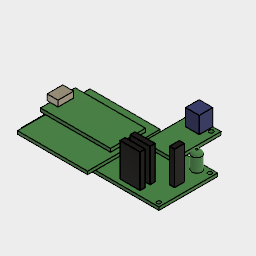
bike_announce_case (Autodesk Fusion 360 archive; units mm, degrees)
design "PCB"
Autodesk Fusion 360 part; units mm, degrees
sketch "Sketch1" plane through (0, 0, 0) normal (0, 0, 1) x (1, 0, 0)
  line L0 (0, 0) -> (70, 0)
  line L1 (70, 0) -> (70, 30)
  line L2 (70, 30) -> (0, 30)
  line L3 (0, 30) -> (0, 0)
  line L4 (0, 15) -> (70, 15) construction
  line L5 (35, 30) -> (35, 0) construction
  circle A0 centre (2, 2) radius 1
  circle A1 centre (2, 28) radius 1
  circle A2 centre (68, 28) radius 1
  circle A3 centre (68, 2) radius 1
  dimension "d1" = 70
  dimension "d2" = 30
  dimension "d22" = 2
  dimension "d23" = 2
  dimension "d24" = 2
  measures "d1" distance of L1.end L2.end
  measures "d2" distance of L0.start L2.end
  measures "d22" diameter of A0
  measures "d23" distance of L0 A0.centre
  measures "d24" distance of L3 A0.centre
extrude "Extrude1" add sketch "Sketch1" along normal blind 1.6 makes body 1
sketch "Sketch5" plane through (0, 0, 1.6) normal (0, 0, 1) x (-1, 0, 0)
  circle A0 centre (-68, -2) radius 1
  circle A1 centre (-2, -2) radius 1
  circle A2 centre (-68, -28) radius 1
  circle A3 centre (-2, -28) radius 1
  line L0 (0, -30) -> (0, 0)
  line L1 (0, 0) -> (-70, 0)
  line L2 (-70, 0) -> (-70, -30)
  line L3 (-70, -30) -> (0, -30)
  line L4 (-47.75, -10.08) -> (-58, -10.08)
  line L5 (-58, -10.08) -> (-58, -7.48)
  line L6 (-58, -7.48) -> (-47.75, -7.48)
  line L7 (-47.75, -7.48) -> (-47.75, -10.08)
  line L8 (-47.75, -5) -> (-58, -5)
  line L9 (-58, -5) -> (-58, -2.4)
  line L10 (-58, -2.4) -> (-47.75, -2.4)
  line L11 (-47.75, -2.4) -> (-47.75, -5)
  line L12 (-58, -3.7) -> (-47.75, -3.7) construction
  line L13 (-47.75, -8.78) -> (-58, -8.78) construction
  line L14 (-62.9, -17.55) -> (-65.5, -17.55)
  line L15 (-65.5, -17.55) -> (-65.5, -12.45)
  line L16 (-65.5, -12.45) -> (-62.9, -12.45)
  line L17 (-62.9, -12.45) -> (-62.9, -17.55)
  line L18 (-62.9, -15) -> (-65.5, -15) construction
  circle A4 centre (-63, -26.3) radius 2.5
  dimension "d25" = 2.6
  dimension "d26" = 10.25
  dimension "d27" = 5.08
  dimension "d28" = 3.7
  dimension "d29" = 12
  dimension "d30" = 2.6
  dimension "d31" = 5.1
  dimension "d32" = 4.5
  dimension "d35" = 5
  dimension "d36" = 3.7
  dimension "d37" = 7
  measures "d25" distance of L4.end L5.end
  measures "d26" distance of L4.start L4.end
  measures "d27" distance of L12 L13
  measures "d28" distance of L1 L12
  measures "d29" distance of L2 L9
  measures "d30" distance of L14.start L14.end
  measures "d31" distance of L14.start L16.end
  measures "d32" distance of L2 L15
  measures "d35" diameter of A4
  measures "d36" distance of L3 A4.centre
  measures "d37" distance of L2 A4.centre
extrude "Extrude5" add sketch "Sketch5" along normal blind 17 separate body contours L4 L5 L6 L7 | L8 L9 L10 L11 | L14 L15 L16 L17 makes body 2 at (51.1667, 10.08, 12.9333) makes body 3 at (51.1667, 5, 12.9333) makes body 4 at (65.5, 15.85, 7.2667)
extrude "Extrude6" add sketch "Sketch5" along normal blind 8.8 separate body contours A4 makes body 5
fillet "Fillet1" radius 2 1 edges at (65.3308, 27.204, 10.4) on bodies 5
ref_plane "WorkPlane1" through (35, 15, 4.1) normal (0, 0, 1) x (1, 0, 0)
sketch "Sketch2" plane through (35, 15, 4.1) normal (0, 0, 1) x (1, 0, 0)
  line L0 (-30.6, 15.5) -> (5.15, 15.5)
  line L1 (5.15, 15.5) -> (5.15, -21.5)
  line L2 (5.15, -21.5) -> (-30.6, -21.5)
  line L3 (-30.6, -21.5) -> (-30.6, 15.5)
  line L4 (-35, 15) -> (-35, -15)
  line L5 (35, 15) -> (-35, 15)
  dimension "d6" = 35.75
  dimension "d7" = 37
  dimension "d8" = 4.4
  dimension "d9" = 0.5
  measures "d6" distance of L0.start L0.end
  measures "d7" distance of L0.start L2.end
  measures "d8" distance of L3 L4
  measures "d9" distance of L0 L5
extrude "Extrude2" add sketch "Sketch2" along normal blind 1.6 separate body makes body 6
ref_plane "WorkPlane2" through (22.275, 12, 8.2) normal (0, 0, 1) x (1, 0, 0)
sketch "Sketch3" plane through (22.275, 12, 8.2) normal (0, 0, 1) x (1, 0, 0)
  line L0 (-17.875, 11) -> (17.875, 11)
  line L1 (17.875, 11) -> (17.875, -6.8)
  line L2 (17.875, -6.8) -> (-17.875, -6.8)
  line L3 (-17.875, -6.8) -> (-17.875, 11)
  line L4 (-17.875, 18.5) -> (-17.875, -18.5)
  line L5 (-17.875, -18.5) -> (-17.875, 18.5)
  line L6 (17.875, -18.5) -> (17.875, 18.5)
  line L7 (17.875, 18.5) -> (17.875, -18.5)
  line L8 (17.875, 18.5) -> (-17.875, 18.5)
  dimension "d13" = 17.8
  dimension "d14" = 7.5
  measures "d13" distance of L0.start L2.end
  measures "d14" distance of L0 L8
extrude "Extrude3" add sketch "Sketch3" along normal blind 1.7 separate body contours L0 L1 L2 L3 L4 L5 L6 L7 makes body 7
sketch "Sketch4" plane through (0, 0, 9.9) normal (0, 0, 1) x (-1, 0, 0)
  line L0 (-4.4, -23) -> (-4.4, -5.2)
  line L1 (-4.4, -5.2) -> (-40.15, -5.2)
  line L2 (-40.15, -5.2) -> (-40.15, -23)
  line L3 (-40.15, -23) -> (-4.4, -23)
  line L4 (-2.9, -18.1) -> (-8.5, -18.1)
  line L5 (-8.5, -18.1) -> (-8.5, -10.1)
  line L6 (-8.5, -10.1) -> (-2.9, -10.1)
  line L7 (-2.9, -10.1) -> (-2.9, -18.1)
  line L8 (-4.4, -14.1) -> (-40.15, -14.1) construction
  dimension "d17" = 5.6
  dimension "d18" = 8
  dimension "d19" = 1.5
  measures "d17" distance of L4.start L4.end
  measures "d18" distance of L4.end L5.end
  measures "d19" distance of L0 L7
extrude "Extrude4" add sketch "Sketch4" along normal blind 3 separate body contours L0 L4 L5 L6 | L0 L4 L6 L7 makes body 8
sketch "Sketch6" plane through (35, 15, 4.1) normal (0, 0, 1) x (1, 0, 0)
  line L0 (6.35, 30) -> (21.7, 30)
  line L1 (21.7, 30) -> (21.7, 5.8)
  line L2 (21.7, 5.8) -> (6.35, 5.8)
  line L3 (6.35, 5.8) -> (6.35, 30)
  circle A0 centre (8.85, 27.5) radius 1.075
  line L4 (14.025, 30) -> (14.025, 5.8) construction
  circle A1 centre (19.2, 27.5) radius 1.075
  line L5 (35, -15) -> (35, 15)
  line L6 (35, 15) -> (-35, 15)
  dimension "d41" = 24.2
  dimension "d42" = 15.35
  dimension "d43" = 2.15
  dimension "d44" = 2.5
  dimension "d45" = 2.5
  dimension "d52" = 13.3
  dimension "d53" = 12.5
  measures "d41" distance of L0.end L1.end
  measures "d42" distance of L0.start L0.end
  measures "d43" diameter of A0
  measures "d44" distance of L3 A0.centre
  measures "d45" distance of L0 A0.centre
  measures "d52" distance of L1 L5
  measures "d53" distance of A1.centre L6
extrude "Extrude7" add sketch "Sketch6" along normal blind 1.65 separate body makes body 9
sketch "Sketch7" plane through (0, 0, 5.75) normal (0, 0, 1) x (-1, 0, 0)
  circle A0 centre (-54.2, -42.5) radius 1.075
  circle A1 centre (-43.85, -42.5) radius 1.075
  line L0 (-41.35, -20.8) -> (-56.7, -20.8)
  line L1 (-56.7, -20.8) -> (-56.7, -45)
  line L2 (-56.7, -45) -> (-41.35, -45)
  line L3 (-41.35, -45) -> (-41.35, -20.8)
  line L4 (-45.525, -45) -> (-52.525, -45)
  line L5 (-52.525, -45) -> (-52.525, -38)
  line L6 (-52.525, -38) -> (-45.525, -38)
  line L7 (-45.525, -38) -> (-45.525, -45)
  line L8 (-49.025, -45) -> (-49.025, -38) construction
  dimension "d48" = 7
  dimension "d49" = 7
  measures "d48" distance of L4.start L4.end
  measures "d49" distance of L4.end L5.end
extrude "Extrude8" add sketch "Sketch7" along normal blind 8.5 separate body contours L2 L4 L5 L6 L7 makes body 10
equation "d27 = ( 2.54 * 2 ) * 1 mm"
named bodies: "Main PCB", "Audio PCB", "Teensy 3.1", "uUSB", "RGB LED Header", "Touch Header", "Power Header", "Green LED", "Amp PCB", "Amp Terminal"

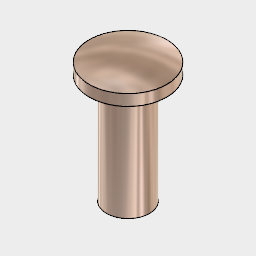
design "touch button"
Autodesk Fusion 360 part; units mm, degrees
sketch "Sketch1" plane through (0, 0, 0) normal (0, 1, 0) x (1, 0, 0)
  line L0 (0, 0) -> (2.8, 0)
  line L1 (2.8, 0) -> (2.8, -1.25)
  line L2 (2.8, -1.25) -> (0, -1.25)
  line L3 (0, -1.25) -> (0, 0)
  line L4 (0, 0) -> (1.55, 0)
  line L5 (1.55, 0) -> (1.55, 7.9)
  line L6 (1.55, 7.9) -> (0, 7.9)
  line L7 (0, 7.9) -> (0, 0)
  arc A0 (-2.8, -0.8) -> (2.8, -0.8) centre (0, 7.6861) ccw
  line L8 (2.8, -0.8) -> (-2.8, -0.8)
  dimension "d1" = 3.1
  dimension "d2" = 5.6
  dimension "d3" = 7.9
  dimension "d4" = 1.25
  dimension "d5" = 0.8
  measures "d3" distance of L4.end L5.end
  measures "d4" distance of L0.end L1.end
  measures "d5" distance of L0 L8
revolve "Revolve1" add sketch "Sketch1" angle 360 about axis through (0, 0, -7.9) along (0, 0, 1) contours L0 L4 L5 L6 L7 | L0 L1 L3 L4 L8 | L3 A0 L8 picked at (0.3158, -1.0832)

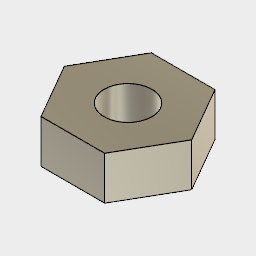
design "clamp nut"
Autodesk Fusion 360 part; units mm, degrees
sketch "Sketch1" plane through (0, 0, 0) normal (0, 0, 1) x (1, 0, 0)
  circle A0 centre (0, 0) radius 3.125 construction
  line L0 (0, 0) -> (0, 3.125) construction
  circle A1 centre (0, 0) radius 1.35
  line L1 (-1.8042, 3.125) -> (-3.6084, 0)
  line L2 (-3.6084, 0) -> (-1.8042, -3.125)
  line L3 (-1.8042, -3.125) -> (1.8042, -3.125)
  line L4 (1.8042, -3.125) -> (3.6084, 0)
  line L5 (3.6084, 0) -> (1.8042, 3.125)
  line L6 (1.8042, 3.125) -> (-1.8042, 3.125)
  dimension "d1" = 6.25
  dimension "d3" = 2.7
  measures "d1" diameter of A0
  measures "d3" diameter of A1
extrude "Extrude1" add sketch "Sketch1" along normal blind 2.45

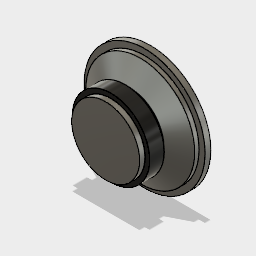
design "speaker"
Autodesk Fusion 360 part; units mm, degrees
sketch "Sketch1" plane through (0, 0, 0) normal (0, 1, 0) x (1, 0, 0)
  line L0 (0, 0) -> (1.1473, 0)
  line L1 (1.1473, 0) -> (25, 0)
  line L2 (25, 0) -> (25, -2.4)
  line L3 (25, -2.4) -> (22.5, -2.4)
  line L4 (22.5, -2.4) -> (22.5, -4.2)
  line L5 (22.5, -4.2) -> (14.05, -8.5)
  line L6 (14.05, -8.5) -> (14.05, -18.5)
  line L7 (14.05, -18.5) -> (0, -18.5)
  line L8 (0, -18.5) -> (0, 0)
  line L9 (14.05, -16.3) -> (16, -16.3)
  line L10 (16, -16.3) -> (16, -10.3)
  line L11 (16, -10.3) -> (14.05, -10.3)
  line L12 (14.05, -10.3) -> (14.05, -16.3)
  dimension "d53" = 50
  dimension "d54" = 2.4
  dimension "d55" = 2.5
  dimension "d56" = 1.8
  dimension "d57" = 28.1
  dimension "d58" = 10
  dimension "d59" = 18.5
  dimension "d60" = 32
  dimension "d61" = 2.2
  dimension "d62" = 6
  dimension "d137" = 0
  dimension "d138" = 0
  dimension "d139" = 0
  dimension "d140" = 0
  dimension "d166" = 0
  dimension "d167" = 0
  dimension "d168" = 0
  dimension "d169" = 0
  dimension "d175" = 0
  dimension "d176" = 0
  dimension "d177" = 0
  dimension "d178" = 0
  dimension "d183" = 0
  dimension "d184" = 0
  dimension "d185" = 0
  dimension "d186" = 0
  measures "d54" distance of L1.end L2.end
  measures "d55" distance of L2.end L3.end
  measures "d56" distance of L3.end L4.end
  measures "d58" distance of L5.end L6.end
  measures "d59" distance of L7.end L0.start
  measures "d61" distance of L6.end L9
  measures "d62" distance of L9.end L10.end
revolve "Revolve1" add sketch "Sketch1" angle 360 about axis through (0, 0, 18.5) along (0, 0, -1)
named bodies: "speaker"

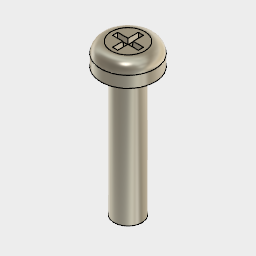
design "clamp bolt"
Autodesk Fusion 360 part; units mm, degrees
sketch "Sketch1" plane through (0, 0, 0) normal (0, 1, 0) x (1, 0, 0)
  line L0 (0, 0) -> (2.625, 0)
  line L1 (2.625, 0) -> (2.625, -2.1)
  line L2 (2.625, -2.1) -> (0, -2.1)
  line L3 (0, -2.1) -> (0, 0)
  line L4 (0, 0) -> (1.35, 0)
  line L5 (1.35, 0) -> (1.35, 12.45)
  line L6 (1.35, 12.45) -> (0, 12.45)
  line L7 (0, 12.45) -> (0, 0)
  dimension "d1" = 2.7
  dimension "d2" = 5.25
  dimension "d3" = 2.1
  dimension "d4" = 12.45
  measures "d3" distance of L0.end L1.end
  measures "d4" distance of L4.end L5.end
revolve "Revolve1" add sketch "Sketch1" angle 360 about axis through (0, 0, 1.75) along (0, 0, 1)
fillet "Fillet1" radius 1 1 edges at (-2.4474, -0.9492, 2.1)
sketch "Sketch2" plane through (0, 0, 2.1) normal (0, 0, 1) x (-1, 0, 0)
  circle A0 centre (0, 0) radius 1.625
  line L0 (0, 0) -> (-1.25, 0)
  line L1 (-1.25, 0) -> (-1.25, -0.25)
  line L2 (-1.25, -0.25) -> (0, -0.25)
  line L3 (0, -0.25) -> (0, 0)
  line L4 (-1.25, 0.25) -> (0, 0.25)
  line L5 (-1.25, 0) -> (-1.25, 0.25)
  line L6 (-0.25, -1.25) -> (-0.25, 0)
  line L7 (0, -1.25) -> (-0.25, -1.25)
  line L8 (0, -1.25) -> (0.25, -1.25)
  line L9 (0.25, -1.25) -> (0.25, 0)
  line L10 (1.25, -0.25) -> (0, -0.25)
  line L11 (1.25, 0) -> (1.25, -0.25)
  line L12 (1.25, 0) -> (1.25, 0.25)
  line L13 (1.25, 0.25) -> (0, 0.25)
  line L14 (0.25, 1.25) -> (0.25, 0)
  line L15 (0, 1.25) -> (0.25, 1.25)
  line L16 (0, 1.25) -> (-0.25, 1.25)
  line L17 (-0.25, 1.25) -> (-0.25, 0)
  dimension "d7" = 0.5
  dimension "d8" = 2.5
  dimension "d10" = 360
extrude "Extrude1" cut sketch "Sketch2" against normal blind 0.5 draft -5 contours L0 L2 L3 L6 | L0 L3 L4 L9 L10 L13 L14 L17 | L0 L1 L2 L6 | L0 L4 L5 L17 | L2 L6 L7 L8 L9 L10 | L4 L13 L14 L15 L16 L17 | L9 L10 L11 L12 L13 L14

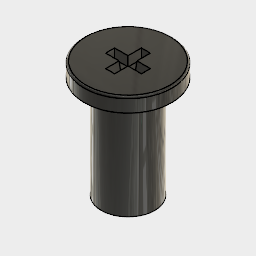
design "case screw"
Autodesk Fusion 360 part; units mm, degrees
sketch "Sketch1" plane through (0, 0, 0) normal (0, 1, 0) x (1, 0, 0)
  line L0 (0, 0) -> (2.45, 0)
  line L1 (2.45, 0) -> (2.45, -0.8)
  line L2 (2.45, -0.8) -> (0, -0.8)
  line L3 (0, -0.8) -> (0, 0)
  line L4 (0, 0) -> (1.495, 0)
  line L5 (1.495, 0) -> (1.495, 5.7)
  line L6 (1.495, 5.7) -> (0, 5.7)
  line L7 (0, 5.7) -> (0, 0)
  dimension "d1" = 4.9
  dimension "d2" = 2.99
  dimension "d3" = 5.7
  dimension "d4" = 0.8
  measures "d3" distance of L4.end L5.end
  measures "d4" distance of L0.end L1.end
revolve "Revolve1" add sketch "Sketch1" angle 360 about axis through (0, 0, 1.75) along (0, 0, 1)
fillet "Fillet1" radius 0.1 1 edges at (-2.2842, -0.886, 0.8)
sketch "Sketch2" plane through (0, 0, 0.8) normal (0, 0, 1) x (-1, 0, 0)
  circle A0 centre (0, 0) radius 2.35
  line L0 (0, 0) -> (-1, 0)
  line L1 (-1, 0) -> (-1, 0.25)
  line L2 (-1, 0.25) -> (0, 0.25)
  line L3 (0, 0.25) -> (0, 0)
  line L4 (-1, 0) -> (-1, -0.25)
  line L5 (-1, -0.25) -> (0, -0.25)
  line L6 (0, -0.25) -> (0, 0)
  line L7 (-0.25, -1) -> (-0.25, 0)
  line L8 (0, -1) -> (0.25, -1)
  line L9 (0, -1) -> (-0.25, -1)
  line L10 (0.25, -1) -> (0.25, 0)
  line L11 (1, -0.25) -> (0, -0.25)
  line L12 (1, 0) -> (1, 0.25)
  line L13 (1, 0) -> (1, -0.25)
  line L14 (1, 0.25) -> (0, 0.25)
  line L15 (0.25, 1) -> (0.25, 0)
  line L16 (0, 1) -> (-0.25, 1)
  line L17 (0, 1) -> (0.25, 1)
  line L18 (-0.25, 1) -> (-0.25, 0)
  dimension "d7" = 0.5
  dimension "d8" = 2
  dimension "d10" = 360
extrude "Extrude1" cut sketch "Sketch2" against normal blind 0.5 draft -5 contours L0 L5 L6 L7 | L0 L2 L3 L18 | L3 L6 L10 L11 L14 L15 | L0 L4 L5 L7 | L0 L1 L2 L18 | L2 L14 L15 L16 L17 L18 | L5 L7 L8 L9 L10 L11 | L10 L11 L12 L13 L14 L15

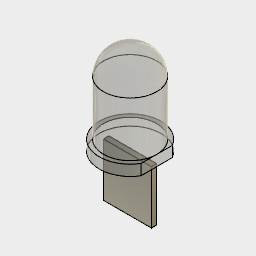
design "RGB LED"
Autodesk Fusion 360 part; units mm, degrees
sketch "Sketch1" plane through (0, 0, 0) normal (0, 1, 0) x (1, 0, 0)
  line L0 (0, 0) -> (2.9, 0)
  line L1 (2.9, 0) -> (2.9, -1)
  line L2 (2.9, -1) -> (0, -1)
  line L3 (0, -1) -> (0, 0)
  line L4 (0, -1) -> (2.5, -1)
  line L5 (2.5, -1) -> (2.5, -6.1)
  line L6 (2.5, -6.1) -> (0, -6.1)
  line L7 (0, -6.1) -> (0, -1)
  arc A0 (0, -8.6) -> (2.5, -6.1) centre (0, -6.1) ccw
  line L8 (0, -6.1) -> (0, -8.6)
  dimension "d2" = 5
  dimension "d3" = 5.8
  dimension "d4" = 1
  dimension "d5" = 8.6
  measures "d4" distance of L0.end L1.end
  measures "d5" distance of L0 A0.start
revolve "Revolve1" add sketch "Sketch1" angle 360 about axis through (0, 0, 6.1) along (0, 0, -1) makes body 1
sketch "Sketch2" plane through (0, 0, 0) normal (0, 0, -1) x (1, 0, 0)
  circle A0 centre (0, 0) radius 2.9
  circle A1 centre (0, 0) radius 2.5
  line L0 (2.5, -1.4697) -> (2.5, 1.4697)
  line L1 (0, 0) -> (2.25, 0)
  line L2 (2.25, 0) -> (2.25, 0.25)
  line L3 (2.25, 0.25) -> (0, 0.25)
  line L4 (0, 0.25) -> (0, 0)
  line L5 (2.25, -0.25) -> (0, -0.25)
  line L6 (0, -0.25) -> (0, 0)
  line L7 (2.25, 0) -> (2.25, -0.25)
  line L8 (-2.25, 0.25) -> (0, 0.25)
  line L9 (-2.25, 0) -> (-2.25, 0.25)
  line L10 (-2.25, 0) -> (-2.25, -0.25)
  line L11 (-2.25, -0.25) -> (0, -0.25)
  dimension "d7" = 4.5
  dimension "d8" = 0.5
extrude "Extrude1" cut sketch "Sketch2" against normal through all contours A0 L0 picked at (2.7581, -0.1281) bodies 1
extrude "Extrude2" add sketch "Sketch2" along normal blind 5 separate body contours L1 L2 L3 L4 | L4 L6 L8 L9 L10 L11 | L1 L5 L6 L7 makes body 2
named bodies: "LED_body", "LED_legs"

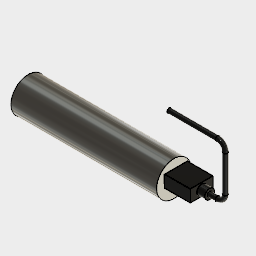
design "usb power bank"
Autodesk Fusion 360 part; units mm, degrees
sketch "Sketch1" plane through (0, 0, 0) normal (1, 0, 0) x (0, 1, 0)
  circle A0 centre (0, 0) radius 10.95
  dimension "d64" = 21.9
  measures "d64" diameter of A0
extrude "Extrude1" add sketch "Sketch1" along normal blind 92.1 makes body 1
sketch "Sketch2" plane through (92.1, 0, 0) normal (1, 0, 0) x (0, 1, 0)
  circle A0 centre (0, 0) radius 10.95
  line L0 (-6.25, 5.35) -> (6.25, 5.35)
  line L1 (6.25, 5.35) -> (6.25, 0.35)
  line L2 (6.25, 0.35) -> (-6.25, 0.35)
  line L3 (-6.25, 0.35) -> (-6.25, 5.35)
  line L4 (-3.625, -2.4) -> (3.625, -2.4)
  line L5 (3.625, -2.4) -> (3.625, -4.65)
  line L6 (3.625, -4.65) -> (-3.625, -4.65)
  line L7 (-3.625, -4.65) -> (-3.625, -2.4)
  line L8 (0, -10.95) -> (0, 10.95) construction
  dimension "d67" = 12.5
  dimension "d68" = 5
  dimension "d69" = 5.6
  dimension "d70" = 7.25
  dimension "d71" = 2.25
  dimension "d72" = 2.75
  measures "d67" distance of L0.start L0.end
  measures "d68" distance of L0.end L1.end
  measures "d69" distance of L0 L8.end
  measures "d70" distance of L5.end L6.end
  measures "d71" distance of L4.end L5.end
  measures "d72" distance of L2 L4
extrude "Extrude2" cut sketch "Sketch2" against normal blind 14 contours L0 L1 L2 L3 | L4 L5 L6 L7 bodies 1
sketch "Sketch3" plane through (92.1, 0, 0) normal (1, 0, 0) x (0, 1, 0)
  line L0 (6.25, 5.35) -> (6.25, 0.35)
  line L1 (6.25, 0.35) -> (-6.25, 0.35)
  line L2 (-6.25, 0.35) -> (-6.25, 5.35)
  line L3 (-6.25, 5.35) -> (6.25, 5.35)
  line L4 (3.625, -2.4) -> (3.625, -4.65)
  line L5 (3.625, -4.65) -> (-3.625, -4.65)
  line L6 (-3.625, -4.65) -> (-3.625, -2.4)
  line L7 (-3.625, -2.4) -> (3.625, -2.4)
  circle A0 centre (0, 0) radius 10.95
  line L8 (-6.025, 5.1) -> (6.025, 5.1)
  line L9 (6.025, 5.1) -> (6.025, 0.6)
  line L10 (6.025, 0.6) -> (-6.025, 0.6)
  line L11 (-6.025, 0.6) -> (-6.025, 5.1)
  line L12 (-6.25, 2.85) -> (6.25, 2.85) construction
  line L13 (0, 0.35) -> (0, 5.35) construction
  dimension "d75" = 12.05
  dimension "d76" = 4.5
  measures "d75" distance of L8.start L8.end
  measures "d76" distance of L8.end L9.end
extrude "Extrude3" add sketch "Sketch3" along normal blind 1.3 separate body contours L8 L9 L10 L11 makes body 2
sketch "Sketch4" plane through (93.4, 0, 0) normal (1, 0, 0) x (0, 1, 0)
  line L0 (-6.025, 0.6) -> (6.025, 0.6)
  line L1 (6.025, 0.6) -> (6.025, 5.1)
  line L2 (6.025, 5.1) -> (-6.025, 5.1)
  line L3 (-6.025, 5.1) -> (-6.025, 0.6)
  line L4 (-7.225, 6.7) -> (7.225, 6.7)
  line L5 (7.225, 6.7) -> (7.225, -1)
  line L6 (7.225, -1) -> (-7.225, -1)
  line L7 (-7.225, -1) -> (-7.225, 6.7)
  line L8 (-6.25, 5.35) -> (6.25, 5.35)
  line L9 (6.25, 0.35) -> (-6.25, 0.35)
  line L10 (0, 5.35) -> (0, 0.35) construction
  line L11 (-6.25, 0.35) -> (-6.25, 5.35)
  line L12 (6.25, 5.35) -> (6.25, 0.35)
  line L13 (-6.25, 2.85) -> (6.25, 2.85) construction
  dimension "d79" = 14.45
  dimension "d80" = 7.7
  measures "d79" distance of L4.start L4.end
  measures "d80" distance of L4.end L5.end
extrude "Extrude4" add sketch "Sketch4" along normal blind 16.25 contours L0 L1 L2 L3 | L4 L5 L6 L7 | L8 L9 L11 L12 bodies 2
sketch "Sketch5" plane through (109.65, 0, 0) normal (1, 0, 0) x (0, 1, 0)
  line L0 (0, 5.35) -> (0, 0.35) construction
  line L1 (-6.25, 2.85) -> (6.25, 2.85) construction
  circle A0 centre (0, 2.85) radius 3.05
  line L2 (-7.225, -1) -> (7.225, -1)
  line L3 (7.225, -1) -> (7.225, 6.7)
  line L4 (7.225, 6.7) -> (-7.225, 6.7)
  line L5 (-7.225, 6.7) -> (-7.225, -1)
  dimension "d83" = 6.1
  measures "d83" diameter of A0
extrude "Extrude5" add sketch "Sketch5" along normal blind 5 contours A0 bodies 2
sketch "Sketch6" plane through (114.65, 0, 0) normal (1, 0, 0) x (0, 1, 0)
  circle A0 centre (0, 2.85) radius 3.05
  circle A1 centre (0, 2.85) radius 1.475
  dimension "d86" = 2.95
  measures "d86" diameter of A1
extrude "Extrude6" add sketch "Sketch6" along normal blind 5 contours A1 bodies 2
move_face "OffsetFaces1" offset 10.95 1 faces at (92.1, 2.0083, 2.1) on bodies 2
sketch "Sketch7" plane through (92.1, 0, 0) normal (1, 0, 0) x (0, 1, 0)
  line L0 (6.25, 5.35) -> (6.25, 0.35)
  line L1 (6.25, 0.35) -> (-6.25, 0.35)
  line L2 (-6.25, 0.35) -> (-6.25, 5.35)
  line L3 (-6.25, 5.35) -> (6.25, 5.35)
  line L4 (3.625, -2.4) -> (3.625, -4.65)
  line L5 (3.625, -4.65) -> (-3.625, -4.65)
  line L6 (-3.625, -4.65) -> (-3.625, -2.4)
  line L7 (-3.625, -2.4) -> (3.625, -2.4)
  circle A0 centre (0, 0) radius 10.95
  line L8 (-11.8424, -1.6) -> (11.8424, -1.6)
  line L9 (-7.225, -1) -> (7.225, -1)
  circle A1 centre (0, 0) radius 11.95
  dimension "d90" = 1
  dimension "d91" = 0.6
  measures "d91" distance of L8 L9
ref_plane "WorkPlane1" through (101.525, 0, 2.85) normal (0, -1, 0) x (0, 0, -1)
sketch "Sketch11" plane through (101.525, 0, 2.85) normal (0, -1, 0) x (0, 0, -1)
  line L0 (1.475, 18.125) -> (-1.475, 18.125)
  line L1 (-5, 23.125) -> (-28, 23.125)
  arc A0 (0, 18.125) -> (-5, 23.125) centre (-5, 18.125) ccw
  line L2 (0, 18.125) -> (0, 23.7232) construction
  line L3 (-33, 18.125) -> (-33, -12.425)
  line L4 (-8.1854, -9.425) -> (-41.003, -9.425) construction
  arc A1 (-28, 23.125) -> (-33, 18.125) centre (-28, 18.125) ccw
  point P0 (0, 18.125)
  dimension "d7" = 5
  dimension "d8" = 23
  dimension "d9" = 5
  dimension "d10" = 3
  measures "d7" radius of A0
  measures "d8" distance of L1.start L1.end
  measures "d9" radius of A1
  measures "d10" distance of L3.end L4
sweep "Sweep1" add 1 faces at (119.65, 0.7495, 2.5324) path "Sketch11" along A0 L1 A1 L3 on bodies 2 bodies 2
equation "d77 = 1.3 mm"
equation "d89 = 12.25 mm - d77"
equation "d8 = 28 mm - 5 mm"
named bodies: "battery", "USB Plug"

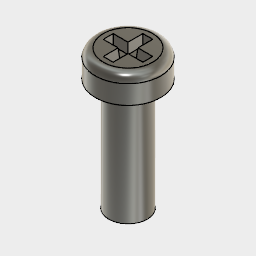
design "pcb screw"
Autodesk Fusion 360 part; units mm, degrees
sketch "Sketch1" plane through (0, 0, 0) normal (0, 1, 0) x (1, 0, 0)
  line L0 (0, 0) -> (1.65, 0)
  line L1 (1.65, 0) -> (1.65, -1.35)
  line L2 (1.65, -1.35) -> (0, -1.35)
  line L3 (0, -1.35) -> (0, 0)
  line L4 (0, 0) -> (0.975, 0)
  line L5 (0.975, 0) -> (0.975, 5.65)
  line L6 (0.975, 5.65) -> (0, 5.65)
  line L7 (0, 5.65) -> (0, 0)
  dimension "d1" = 3.3
  dimension "d2" = 1.35
  dimension "d3" = 1.95
  dimension "d4" = 5.65
  measures "d2" distance of L0.end L1.end
  measures "d4" distance of L4.end L5.end
revolve "Revolve1" add sketch "Sketch1" angle 360 about axis through (0, 0, -5.65) along (0, 0, 1)
fillet "Fillet1" radius 0.4 1 edges at (-1.5383, -0.5967, 1.35)
sketch "Sketch2" plane through (0, 0, 1.35) normal (0, 0, 1) x (-1, 0, 0)
  circle A0 centre (0, 0) radius 1.25
  line L0 (0, 0) -> (-1, 0)
  line L1 (-1, 0) -> (-1, 0.25)
  line L2 (-1, 0.25) -> (0, 0.25)
  line L3 (0, 0.25) -> (0, 0)
  line L4 (-1, 0) -> (-1, -0.25)
  line L5 (-1, -0.25) -> (0, -0.25)
  line L6 (0, -0.25) -> (0, 0)
  line L7 (0.25, -1) -> (0.25, 0)
  line L8 (0, -1) -> (0.25, -1)
  line L9 (0, -1) -> (-0.25, -1)
  line L10 (-0.25, -1) -> (-0.25, 0)
  line L11 (1, 0.25) -> (0, 0.25)
  line L12 (1, 0) -> (1, 0.25)
  line L13 (1, 0) -> (1, -0.25)
  line L14 (1, -0.25) -> (0, -0.25)
  line L15 (-0.25, 1) -> (-0.25, 0)
  line L16 (0, 1) -> (-0.25, 1)
  line L17 (0, 1) -> (0.25, 1)
  line L18 (0.25, 1) -> (0.25, 0)
  dimension "d7" = 0.5
  dimension "d8" = 2
  dimension "d10" = 360
extrude "Extrude1" cut sketch "Sketch2" against normal blind 0.5 draft -5 contours L0 L5 L6 L10 | L0 L2 L3 L15 | L3 L6 L7 L11 L14 L18 | L0 L4 L5 L10 | L0 L1 L2 L15 | L2 L11 L15 L16 L17 L18 | L5 L7 L8 L9 L10 L14 | L7 L11 L12 L13 L14 L18

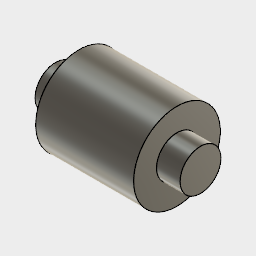
design "center handle bar"
Autodesk Fusion 360 part; units mm, degrees
sketch "Sketch1" plane through (0, 0, 0) normal (1, 0, 0) x (0, 1, 0)
  circle A0 centre (0, 0) radius 23
  circle A1 centre (0, 0) radius 10.875
  dimension "d1" = 46
  dimension "d2" = 21.75
  measures "d1" diameter of A0
  measures "d2" diameter of A1
extrude "Extrude1" add sketch "Sketch1" along normal mid plane 52 contours A0 | A1
extrude "Extrude2" add sketch "Sketch1" along normal mid plane 77 contours A1

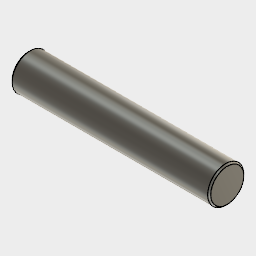
design "clamp pin"
Autodesk Fusion 360 part; units mm, degrees
sketch "Sketch1" plane through (0, 0, 0) normal (1, 0, 0) x (0, 1, 0)
  circle A0 centre (0, 0) radius 1.185
  dimension "d1" = 2.37
  measures "d1" diameter of A0
extrude "Extrude1" add sketch "Sketch1" along normal blind 13
chamfer "Chamfer1" distance 0.1 angle 45 2 edges at (13, -1.1048, -0.4285) (0, -1.1048, -0.4285)
